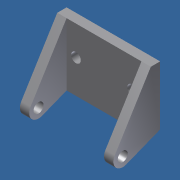
# Autodesk Inventor part: kinect bracket b
Saved by Autodesk Inventor 2012 (Build 160160000, 160)
## iProperties
Created: 2012-10-30
Part Number: kinect bracket b
Material: Default
Document SubType Name: Modeling
Designer: Ed
Density: 1 g/cm^3
Author: Ed
Autodesk Inventor part; units mm, degrees
ref_plane "YZ Plane" through (0, 0, 0) normal (1, 0, 0) x (0, 1, 0)
ref_plane "XZ Plane" through (0, 0, 0) normal (0, 1, 0) x (-1, 0, 0)
ref_plane "XY Plane" through (0, 0, 0) normal (0, 0, 1) x (1, 0, 0)
sketch "Sketch1" plane through (0, 0, 0) normal (0, 0, 1) x (1, 0, 0)
  line L0 (0, 0) -> (63.5, 0)
  line L1 (63.5, 0) -> (63.5, 40)
  line L2 (63.5, 40) -> (0, 40)
  line L3 (0, 40) -> (0, 0)
  dimension "d2" = 40
  dimension "d3" = 63.5
  constraints: 8 end point, 2 parallel, 1 horizontal, 1 perpendicular
  measures "d2" distance of L2.end L0.start
  measures "d3" distance of L0.start L0.end
extrude "Extrusion1" add sketch "Sketch1" along normal blind 6.35
sketch "Sketch2" plane through (0, 0, 6.35) normal (0, 0, 1) x (1, 0, 0)
  line L0 (0, 0) -> (0, 40) projected
  line L1 (0, 40) -> (63.5, 40) projected
  line L2 (50.8, 20) -> (12.7, 20)
  point P0 (0, 20)
  point P1 (31.75, 20)
  point P2 (31.75, 40)
  dimension "d4" = 38.1
  constraints: 3 midpoint, 2 end point, 2 horizontal alignment, 1 parallel, 1 vertical alignment
  measures "d4" distance of L2.start L2.end
hole "Hole1" at (12.7, 20, 6.35) at (50.8, 20, 6.35) direction (0, 0, -1) diameter 6.604 end through all clearance for "Flat Head Machine Screw" size "M6" standard "Ansi Metric M Profile"
sketch "Sketch3" plane through (63.5, 0, 0) normal (1, 0, 0) x (0, 0, -1)
  line L0 (-6.35, 40) -> (-6.35, 0) projected
  line L1 (0, 0) -> (-6.35, 0) projected
  line L2 (0, 0) -> (0, 40) projected
  circle A0 centre (-25.4, -3.175) radius 6.35
  line L3 (0, 0) -> (-23.0739, -9.0836)
  line L4 (-30.8119, 0.1468) -> (-6.35, 40)
  dimension "d12" = 12.7
  dimension "d13" = 3.175
  dimension "d14" = 25.4
  constraints: 4 end point, 2 point on circle, 2 tangent, 1 centre point
  measures "d12" diameter of A0
  measures "d13" distance from line of L1 A0.centre
  measures "d14" distance from line of L2 A0.centre
extrude "Extrusion2" add sketch "Sketch3" against normal up to surface (63.5 mm away)
sketch "Sketch4" plane through (0, 40, 0) normal (0, 1, 0) x (1, 0, 0)
  line L0 (0, -6.35) -> (63.5, -6.35) projected
  line L1 (63.5, 0) -> (63.5, -6.35) projected
  line L2 (0, 0) -> (0, -6.35) projected
  line L3 (6.35, -6.35) -> (57.15, -6.35)
  line L4 (57.15, -6.35) -> (57.15, -38.1)
  line L5 (57.15, -38.1) -> (6.35, -38.1)
  line L6 (6.35, -38.1) -> (6.35, -6.35)
  dimension "d17" = 31.75
  dimension "d18" = 6.35
  dimension "d19" = 6.35
  constraints: 8 end point, 2 parallel, 1 horizontal, 1 perpendicular, 1 point on line
  measures "d17" distance between parallel lines of L3 L5
  measures "d18" distance between parallel lines of L1 L4
  measures "d19" distance between parallel lines of L2 L6
extrude "Extrusion3" cut sketch "Sketch4" against normal through all
hole "Hole2" at (63.5, -3.175, 25.4) direction (-1, 0, 0) diameter 6.7564 end through all clearance for "Flat Head Machine Screw (82)" size "1/4" standard "Ansi Unified Screw Threads"
body "Solid1"
